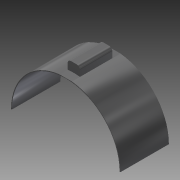
# Autodesk Inventor part: Drill Motor Shifter Cover
Saved by Autodesk Inventor 2012 (Build 160160000, 160)
## iProperties
Created: 2012-07-04
Part Number: Drill Motor Shifter Cover
Material: Default
Document SubType Name: Modeling
Designer: Bruce
Density: 1 g/cm^3
Author: Bruce
Autodesk Inventor part; units mm, degrees
ref_plane "YZ Plane" through (0, 0, 0) normal (1, 0, 0) x (0, 1, 0)
ref_plane "XZ Plane" through (0, 0, 0) normal (0, 1, 0) x (-1, 0, 0)
ref_plane "XY Plane" through (0, 0, 0) normal (0, 0, 1) x (1, 0, 0)
sketch "Sketch1" plane through (0, 0, 0) normal (0, 0, 1) x (1, 0, 0)
  arc A0 (25.7556, 0) -> (-16.846658, 19.481813) centre (0, 0) ccw
  arc A1 (-16.846658, 19.481813) -> (-25.7556, 0) centre (0, 0) ccw
  arc A2 (25.4, 0) -> (-25.4, 0) centre (0, 0) ccw
  line L0 (-25.4, 0) -> (-25.7556, 0)
  line L1 (25.4, 0) -> (25.7556, 0)
  line L2 (-2.921, 25.589425) -> (2.921, 25.589425)
  line L3 (2.921, 25.589425) -> (2.921, 29.907425)
  line L4 (2.921, 29.907425) -> (-2.921, 29.907425)
  line L5 (-2.921, 29.907425) -> (-2.921, 25.589425)
  point P0 (25.5778, 0)
  point P1 (-25.5778, 0)
  dimension "d16" = 25.4
  dimension "d18" = 5.842
  dimension "d19" = 2.921
  dimension "d20" = 4.318
  dimension "d23" = 0.3556
  dimension "d24" = 25.7556
  constraints: 12 end point, 9 point on circle, 3 centre point, 3 equal length, 2 horizontal, 2 horizontal alignment, 2 midpoint, 1 coincident, 1 perpendicular
  measures "d16" radius of A2
  measures "d18" distance of L3.end L4.end
  measures "d19" distance from line of L5 point (0, 0)
  measures "d20" distance of L4.end L2.start
  measures "d23" distance of L0.start L0.end
  measures "d24" radius of A0
sketch "Sketch1 outline for Extrusion1" plane through (0, 0, 0) normal (0, 0, 1) x (1, 0, 0)
  line L0 (25.4, 0) -> (25.7556, 0)
  arc A0 (-25.4, 0) -> (25.4, 0) centre (0, 0) cw
  line L1 (-25.7556, 0) -> (-25.4, 0)
  arc A1 (-16.846658, 19.481813) -> (-25.7556, 0) centre (0, 0) ccw
  arc A2 (-2.921, 25.589425) -> (-16.846658, 19.481813) centre (0, 0) ccw
  line L2 (2.921, 25.589425) -> (-2.921, 25.589425)
  arc A3 (25.7556, 0) -> (2.921, 25.589425) centre (0, 0) ccw
extrude "Extrusion1" add sketch "Sketch1 outline for Extrusion1" along normal mid plane 22.86
extrude "Extrusion2" add sketch "Sketch1" along normal mid plane 15.24 contours A0 L5 L4 L3
fillet "Fillet1" radius 1.5875 2 edges at (2.921, 29.9074, 0) (-2.921, 29.9074, 0)
equation "\"d19\" = 0.5 * d18"
equation "\"d24\" = d16 + d23"
body "Solid1"
